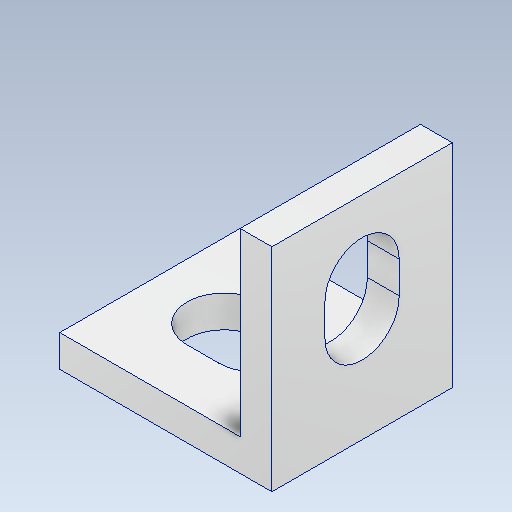
# Autodesk Inventor part: 2020RightAngle
Saved by Autodesk Inventor 2021.1 (Build 251245010, 245A)
## iProperties
Created: 2023-10-30
Part Number: 2020RightAngle
Material: Aluminum 6061
Document SubType Name: Modeling
Designer: M
Density: 2.7 g/cm^3
Appearance: Aluminum - Flat
Author: M
Autodesk Inventor part; units mm, degrees
ref_plane "YZ Plane" through (0, 0, 0) normal (1, 0, 0) x (0, 1, 0)
ref_plane "XZ Plane" through (0, 0, 0) normal (0, 1, 0) x (-1, 0, 0)
ref_plane "XY Plane" through (0, 0, 0) normal (0, 0, 1) x (1, 0, 0)
sketch "Sketch1" plane through (0, 0, 0) normal (1, 0, 0) x (0, 1, 0)
  line L0 (0, 0) -> (20, 0)
  line L1 (20, 0) -> (20, -17)
  line L2 (20, -17) -> (0, -17)
  line L3 (0, -17) -> (0, 0)
  dimension "d0" = 20
  dimension "d1" = 17
  constraints: 8 end point, 2 parallel, 1 horizontal, 1 perpendicular
  measures "d0" distance of L1.end L2.end
  measures "d1" distance of L0.end L1.end
extrude "Extrusion1" add sketch "Sketch1" along normal blind 3
sketch "Sketch2" plane through (0, 0, -17) normal (0, -1, 0) x (1, 0, 0)
  line L0 (3, 0) -> (3, 17) projected
  line L1 (3, 17) -> (-17, 17)
  line L2 (-17, 17) -> (-17, 0)
  line L3 (-17, 0) -> (3, 0)
  line L4 (3, 0) -> (3, 17)
  line L5 (-17, 17) -> (-17, 0)
  line L6 (0, 0) -> (-17, 0)
  line L7 (0, 17) -> (0, 0)
  line L8 (-17, 17) -> (0, 17)
  line L9 (-10, 8.5) -> (-7, 8.5) construction
  line L10 (-10, 5) -> (-7, 5)
  line L11 (-7, 12) -> (-10, 12)
  arc A0 (-10, 12) -> (-10, 5) centre (-10, 8.5) ccw
  arc A1 (-7, 5) -> (-7, 12) centre (-7, 8.5) ccw
  point P0 (0, 17)
  point P1 (0, 0)
  point P2 (-8.5, 8.5)
  dimension "d4" = 20
  dimension "d15" = 7
  dimension "d16" = 3
  dimension "d17" = 7
  dimension "d18" = 17
  dimension "d19" = 17
  dimension "d20" = 8.5
  constraints: 24 end point, 5 parallel, 4 point on circle, 4 tangent, 2 centre point, 2 horizontal, 1 coincident, 1 midpoint, 1 perpendicular, 1 vertical
  measures "d4" distance of L3.end L2.end
  measures "d15" diameter of A1
  measures "d16" distance of L9.start L9.end
  measures "d17" distance from line of L7 L9.end
  measures "d18" distance of L5.start L7.start
  measures "d19" distance of L7.start L6.start
  measures "d20" distance between parallel lines of L6 L9
extrude "Extrusion2" add sketch "Sketch2" against normal blind 3 contours L3 L7 L1 L0 | L3 L2 L1 L7 | A0 L11 A1 L10
sketch "Sketch3" plane through (0, 0, 0) normal (-1, 0, 0) x (0, 0, 1)
  line L0 (-17, 3) -> (0, 3)
  line L1 (0, 20) -> (0, 3)
  line L2 (-17, 20) -> (0, 20)
  line L3 (-17, 3) -> (-17, 20)
  line L4 (-8.5, 10) -> (-8.5, 13) construction
  line L5 (-5, 10) -> (-5, 13)
  line L6 (-12, 13) -> (-12, 10)
  arc A0 (-12, 10) -> (-5, 10) centre (-8.5, 10) ccw
  arc A1 (-5, 13) -> (-12, 13) centre (-8.5, 13) ccw
  point P0 (0, 0)
  point P1 (-8.5, 11.5)
  dimension "d7" = 7
  dimension "d8" = 3
  dimension "d9" = 7
  dimension "d10" = 17
  dimension "d11" = 17
  dimension "d12" = 8.5
  constraints: 16 end point, 4 point on circle, 4 tangent, 3 vertical, 2 centre point, 2 horizontal, 1 midpoint, 1 parallel, 1 other
  measures "d7" diameter of A1
  measures "d8" distance of L4.start L4.end
  measures "d9" distance from line of L2 L4.end
  measures "d10" distance of L0.start L2.start
  measures "d11" distance of L2.start L1.start
  measures "d12" distance between parallel lines of L1 L4
extrude "Extrusion3" cut sketch "Sketch3" against normal blind 3 contours A0 L6 A1 L5
extrude "Extrusion4" cut sketch "Sketch2" against normal blind 3 contours A0 L11 A1 L10
equation "\"d17\" = -0.5 * d16 + 0.5 * d18"
equation "\"d20\" = 0.5 * d19"
equation "\"d9\" = -0.5 * d8 + 0.5 * d10"
equation "\"d12\" = 0.5 * d11"
body "Solid1"
